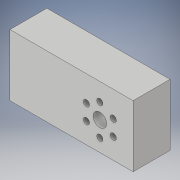
# Autodesk Inventor part: MotorHolderB
Saved by Autodesk Inventor 2017 (Build 210142000, 142)
## iProperties
Created: 2017-12-08
Part Number: MotorHolderB
Material: Generic
Document SubType Name: Modeling
Designer: User
Density: 1 g/cm^3
Appearance: Default
Author: User
Autodesk Inventor part; units mm, degrees
ref_plane "YZ Plane" through (0, 0, 0) normal (1, 0, 0) x (0, 1, 0)
ref_plane "XZ Plane" through (0, 0, 0) normal (0, 1, 0) x (-1, 0, 0)
ref_plane "XY Plane" through (0, 0, 0) normal (0, 0, 1) x (1, 0, 0)
sketch "Sketch1" plane through (0, 0, 0) normal (0, 0, 1) x (1, 0, 0)
  line L0 (0, 0) -> (63.5, 0)
  line L1 (63.5, 0) -> (63.5, 31.75)
  line L2 (63.5, 31.75) -> (0, 31.75)
  line L3 (0, 31.75) -> (0, 0)
  dimension "d0" = 63.5
  dimension "d1" = 31.75
  constraints: 8 end point, 2 parallel, 1 horizontal, 1 perpendicular
  measures "d0" distance of L2.end L1.end
  measures "d1" distance of L1.end L0.end
extrude "Extrusion1" add sketch "Sketch1" along normal blind 19.05
sketch "Sketch2" plane through (0, 0, 19.05) normal (0, 0, 1) x (1, 0, 0)
  line L0 (63.5, 0) -> (63.5, 31.75) projected
  line L1 (63.5, 12.7901) -> (80.6196, 12.7901) construction
  line L2 (0, 0) -> (63.5, 0) projected
  line L3 (46.3804, 0) -> (46.3804, 14.605)
  line L4 (46.3804, 0) -> (60.9854, 0) construction
  circle A0 centre (46.3804, 14.605) radius 3.4925
  circle A1 centre (46.3804, 14.605) radius 8.001
  circle A2 centre (46.3804, 6.604) radius 1.5875
  circle A3 centre (53.3095, 10.6045) radius 1.5875
  circle A4 centre (46.3804, 14.605) radius 8.001
  circle A5 centre (53.3095, 18.6055) radius 1.5875
  circle A6 centre (46.3804, 14.605) radius 8.001
  circle A7 centre (46.3804, 22.606) radius 1.5875
  circle A8 centre (46.3804, 14.605) radius 8.001
  circle A9 centre (39.4513, 18.6055) radius 1.5875
  circle A10 centre (46.3804, 14.605) radius 8.001
  circle A11 centre (39.4513, 10.6045) radius 1.5875
  circle A12 centre (46.3804, 14.605) radius 8.001
  dimension "d9" = 16.002
  dimension "d6" = 14.605
  dimension "d7" = 90
  dimension "d8" = 6.985
  dimension "d10" = 3.175
  dimension "d13" = 360
  constraints: 7 centre point, 6 end point, 3 point on line, 2 coincident, 2 horizontal, 2 perpendicular, 2 vertical alignment, 41 other
  measures "d6" distance of L3.start L3.end
  measures "d7" angle of L4 L3
  measures "d8" diameter of A0
  measures "d10" diameter of A2
extrude "Extrusion2" cut sketch "Sketch2" against normal blind 19.05 contours A2 A1 L3 | L3 A1 A2 | A1 A2 L3 | L3 A2 A1 | A11 A1 | A1 A11 | A3 A1 | A1 A3 | A9 A1 | A1 A9 | A5 A1 | A1 A5 | A7 A1 | A1 A7 | A0
body "Solid1"
